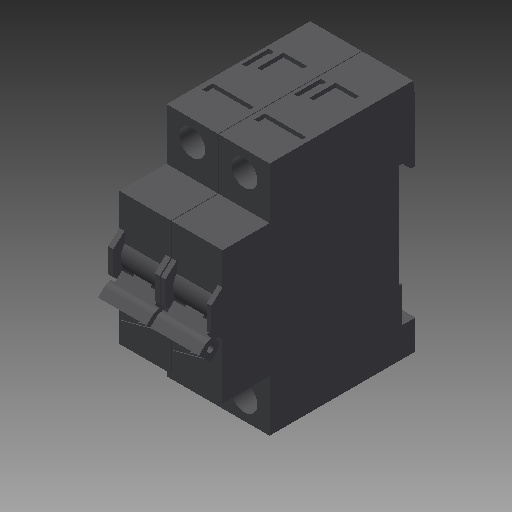
# Autodesk Inventor part: 278738
Saved by Autodesk Inventor 2019.3 (Build 233278000, 278)
## iProperties
Category: PARTsolutions
Company: MOELLER
Created: 2017-12-07
Part Number: 278738
Catalog Web Link: www.cadenas.de
Description: Miniature Circuit Breakers (MCBs)-
Vendor: MOELLER
Document SubType Name: Modeling
Designer: psAdmin
Manufacturer: MOELLER
Mass: 154.066 g
Surface Area: 233.199 cm^2
Volume: 154.066 cm^3
Density: 1 g/cm^3
Material: Типовые
Appearance: PSOLRGB-175-175-175
PSOL_IDENT_0: {$CADENAS_DATA\23d-libs\moeller\36899\36901\36903\36910.prj},196 {VTYP=3D},{NB=278738},{LINA=278738}
PSOL_IDENT_1: ,{NN=Miniature Circuit Breakers (MCBs)},{DATE=03.11.2017 09:05:45},{GEOMDATE=02.11.2017 14:51:53},{V
PSOL_IDENT_2: ERSION=v171102145153},{LINEID=8470},{LINESUBID=-1},{WBVAR=}  {NB=278738},{LINA=278738},{KT=DUMMY},{P
PSOL_IDENT_3: FOTO=sg55112.jpg},{PLID=278738},{DATA_SHEET=Data sheet},{MANUTYPEDESC=FAZ-B40/2},{DESCSHORT=Miniatur
PSOL_IDENT_4: e circuit breaker (MCB), 40A, 2p, B-Char, AC},{DESCLONG=Miniature circuit breaker (MCB) FAZ, 2 pole,
PSOL_IDENT_5: Tripping characteristic: B, Rated current In: 40 A, Switchgear for industrial and advanced commerci
PSOL_IDENT_6: al applications},{EAN=4015082787387},{ECLASS_8_1=27-14-19-01},{PACKAGED_WEIGHT=0.233},{DATA_SHEET_=h
PSOL_IDENT_7: ttp://datasheet.moeller.net/datasheet.php?model=278738&locale=en_GB},{DATA_SHEET_ENG=http://datashee
PSOL_IDENT_8: t.moeller.net/datasheet.php?model=278738&locale=en_GB},{DATA_SHEET_DEU=http://datasheet.moeller.net/
PSOL_IDENT_9: datasheet.php?model=278738&locale=de_DE}
NN: Miniature Circuit Breakers (MCBs)
NB: 278738
NBSYN: $PLID.
LINA: 278738
PFOTO: sg55112.jpg
PLID: 278738
DATA_SHEET: Data sheet
MANUTYPEDESC: FAZ-B40/2
DESCSHORT: Miniature circuit breaker (MCB), 40A, 2p, B-Char, AC
DESCLONG: Miniature circuit breaker (MCB) FAZ, 2 pole, Tripping characteristic: B, Rated current In: 40 A, Switchgear for industrial and advanced commercial applications
EAN: 4015082787387
ECLASS_8_1: 27-14-19-01
PACKAGED_WEIGHT: 0.233
SUPPLIER: MOELLER
ARTICLENO: 278738
BOMINFO: 278738
CREATOR: CADENAS GmbH
Title: 278738
Author: Cadenas PARTsolutions
Autodesk Inventor part; units mm, degrees
ref_plane "YZ Plane" through (0, 0, 0) normal (1, 0, 0) x (0, 1, 0)
ref_plane "XZ Plane" through (0, 0, 0) normal (0, 1, 0) x (-1, 0, 0)
ref_plane "XY Plane" through (0, 0, 0) normal (0, 0, 1) x (1, 0, 0)
sketch "Sketch_1" plane through (8.75, 0, 0) normal (1, 0, 0) x (0, 0, -1)
  line L0 (-63.8, 8.1) -> (-63.8, -0.1)
  line L1 (-63.8, -0.1) -> (-60, -3.6)
  line L2 (-60, -3.6) -> (-60, -22.5)
  line L3 (-60, -22.5) -> (-44, -22.5)
  line L4 (-44, -22.5) -> (-44, -40)
  line L5 (-44, -40) -> (5.5, -40)
  line L6 (5.5, -40) -> (5.5, -30)
  line L7 (5.5, -30) -> (1, -30)
  line L8 (1, -30) -> (1, -18.1)
  arc A0 (1, -18.1) -> (0.7, -17.8) centre (0.7, -18.1) ccw
  line L9 (0.7, -17.8) -> (0, -17.8)
  line L10 (0, -17.8) -> (0, 17.5)
  line L11 (0, 17.5) -> (1, 17.5)
  line L12 (1, 17.5) -> (4, 14.5)
  line L13 (4, 14.5) -> (5.5, 14.5)
  line L14 (5.5, 14.5) -> (5.5, 34)
  line L15 (5.5, 34) -> (4.7633, 40)
  line L16 (4.7633, 40) -> (-44, 40)
  line L17 (-44, 40) -> (-44, 22.5)
  line L18 (-44, 22.5) -> (-60, 22.5)
  line L19 (-60, 22.5) -> (-60, 11.6)
  line L20 (-60, 11.6) -> (-63.8, 8.1)
  constraints: 42 end point, 2 point on circle, 1 centre point
extrude "Extrusion1" add sketch "Sketch_1" along normal mid plane 17.5
sketch "Sketch_5" plane through (0, 0, 0) normal (0, 1, 0) x (-1, 0, 0)
  line L0 (-1.05, 19.5) -> (-2.9801, 19.5)
  line L1 (-2.9801, 19.5) -> (-2.9801, 10.4)
  line L2 (-2.9801, 10.4) -> (-1.05, 10.4)
  line L3 (-1.05, 10.4) -> (-1.05, 19.5)
  constraints: 8 end point
extrude "Extrusion2" cut sketch "Sketch_5" along normal mid plane 100
sketch "Sketch_6" plane through (0, 0, 0) normal (0, 1, 0) x (-1, 0, 0)
  line L0 (-4.75, 18) -> (-12.75, 18)
  line L1 (-12.75, 18) -> (-12.75, 9)
  line L2 (-12.75, 9) -> (-4.75, 9)
  line L3 (-4.75, 9) -> (-4.75, 18)
  constraints: 8 end point
extrude "Extrusion3" cut sketch "Sketch_6" along normal mid plane 100
sketch "Sketch_7" plane through (0, 0, 0) normal (0, 1, 0) x (-1, 0, 0)
  line L0 (-1.75, 33.6) -> (-15.75, 33.6)
  line L1 (-15.75, 33.6) -> (-15.75, 30)
  line L2 (-15.75, 30) -> (-1.75, 30)
  line L3 (-1.75, 30) -> (-1.75, 33.6)
  constraints: 8 end point
extrude "Extrusion4" cut sketch "Sketch_7" along normal mid plane 100
sketch "Sketch_8" plane through (0, 0, 0) normal (0, 1, 0) x (-1, 0, 0)
  line L0 (-0.75, 38) -> (-16.25, 38)
  line L1 (-16.25, 38) -> (-16.25, 8)
  line L2 (-16.25, 8) -> (-0.75, 8)
  line L3 (-0.75, 8) -> (-0.75, 38)
  constraints: 8 end point
extrude "Extrusion5" add sketch "Sketch_8" along normal mid plane 77.2
sketch "Sketch_19" plane through (0, 0, 60) normal (0, 0, 1) x (1, 0, 0)
  line L0 (0.05, -15.4982) -> (14.2251, -11.7)
  line L1 (14.2251, -11.7) -> (0.05, -7.9018)
  line L2 (0.05, -7.9018) -> (0.05, -15.4982)
  constraints: 6 end point
extrude "Extrusion6" cut sketch "Sketch_19" along normal mid plane 0.6
sketch "Sketch_20" plane through (0, 0, 60) normal (0, 0, 1) x (1, 0, 0)
  line L0 (5.95, -13.3345) -> (12.05, -11.7)
  line L1 (12.05, -11.7) -> (5.95, -10.0655)
  line L2 (5.95, -10.0655) -> (5.95, -13.3345)
  constraints: 6 end point
extrude "Extrusion7" cut sketch "Sketch_20" against normal blind 0.8
sketch "Sketch_22" plane through (26.45, 0, 0) normal (1, 0, 0) x (0, 0, -1)
  line L0 (-59.8, -22.3) -> (-43.8, -22.3)
  line L1 (-43.8, -22.3) -> (-43.8, -39.8)
  line L2 (-43.8, -39.8) -> (5.3, -39.8)
  line L3 (5.3, -39.8) -> (5.3, -30.2)
  line L4 (5.3, -30.2) -> (0.8, -30.2)
  line L5 (0.8, -30.2) -> (0.8, -18.3)
  arc A0 (0.8, -18.3) -> (0.5, -18) centre (0.5, -18.3) ccw
  line L6 (0.5, -18) -> (-0.2, -18)
  line L7 (-0.2, -18) -> (-0.2, 17.7)
  line L8 (-0.2, 17.7) -> (1, 17.7)
  line L9 (1, 17.7) -> (4, 14.7)
  line L10 (4, 14.7) -> (5.3, 14.7)
  line L11 (5.3, 14.7) -> (5.3, 34)
  line L12 (5.3, 34) -> (4.5878, 39.8)
  line L13 (4.5878, 39.8) -> (-43.8, 39.8)
  line L14 (-43.8, 39.8) -> (-43.8, 22.3)
  line L15 (-43.8, 22.3) -> (-59.8, 22.3)
  line L16 (-59.8, 22.3) -> (-59.8, -22.3)
  constraints: 34 end point, 2 point on circle, 1 centre point
extrude "Extrusion8" add sketch "Sketch_22" against normal blind 9
sketch "Sketch_24" plane through (26.45, 0, 0) normal (1, 0, 0) x (0, 0, -1)
  line L0 (-63.8, 8.1) -> (-63.8, -0.1)
  line L1 (-63.8, -0.1) -> (-60, -3.6)
  line L2 (-60, -3.6) -> (-60, -22.5)
  line L3 (-60, -22.5) -> (-44, -22.5)
  line L4 (-44, -22.5) -> (-44, -40)
  line L5 (-44, -40) -> (5.5, -40)
  line L6 (5.5, -40) -> (5.5, -30)
  line L7 (5.5, -30) -> (1, -30)
  line L8 (1, -30) -> (1, -18.1)
  arc A0 (1, -18.1) -> (0.7, -17.8) centre (0.7, -18.1) ccw
  line L9 (0.7, -17.8) -> (0, -17.8)
  line L10 (0, -17.8) -> (0, 17.5)
  line L11 (0, 17.5) -> (1, 17.5)
  line L12 (1, 17.5) -> (4, 14.5)
  line L13 (4, 14.5) -> (5.5, 14.5)
  line L14 (5.5, 14.5) -> (5.5, 34)
  line L15 (5.5, 34) -> (4.7633, 40)
  line L16 (4.7633, 40) -> (-44, 40)
  line L17 (-44, 40) -> (-44, 22.5)
  line L18 (-44, 22.5) -> (-60, 22.5)
  line L19 (-60, 22.5) -> (-60, 11.6)
  line L20 (-60, 11.6) -> (-63.8, 8.1)
  constraints: 42 end point, 2 point on circle, 1 centre point
extrude "Extrusion9" add sketch "Sketch_24" along normal mid plane 17.1
sketch "Sketch_28" plane through (0, 0, 0) normal (0, 1, 0) x (-1, 0, 0)
  line L0 (-18.75, 19.5) -> (-20.6801, 19.5)
  line L1 (-20.6801, 19.5) -> (-20.6801, 10.4)
  line L2 (-20.6801, 10.4) -> (-18.75, 10.4)
  line L3 (-18.75, 10.4) -> (-18.75, 19.5)
  constraints: 8 end point
extrude "Extrusion10" cut sketch "Sketch_28" along normal mid plane 100
sketch "Sketch_29" plane through (0, 0, 0) normal (0, 1, 0) x (-1, 0, 0)
  line L0 (-22.45, 18) -> (-30.45, 18)
  line L1 (-30.45, 18) -> (-30.45, 9)
  line L2 (-30.45, 9) -> (-22.45, 9)
  line L3 (-22.45, 9) -> (-22.45, 18)
  constraints: 8 end point
extrude "Extrusion11" cut sketch "Sketch_29" along normal mid plane 100
sketch "Sketch_30" plane through (0, 0, 0) normal (0, 1, 0) x (-1, 0, 0)
  line L0 (-19.45, 33.6) -> (-33.45, 33.6)
  line L1 (-33.45, 33.6) -> (-33.45, 30)
  line L2 (-33.45, 30) -> (-19.45, 30)
  line L3 (-19.45, 30) -> (-19.45, 33.6)
  constraints: 8 end point
extrude "Extrusion12" cut sketch "Sketch_30" along normal mid plane 100
sketch "Sketch_31" plane through (0, 0, 0) normal (0, 1, 0) x (-1, 0, 0)
  line L0 (-18.25, 38) -> (-33.75, 38)
  line L1 (-33.75, 38) -> (-33.75, 8)
  line L2 (-33.75, 8) -> (-18.25, 8)
  line L3 (-18.25, 8) -> (-18.25, 38)
  constraints: 8 end point
extrude "Extrusion13" add sketch "Sketch_31" along normal mid plane 77.2
sketch "Sketch_13" plane through (0, 0, 0) normal (0, 1, 0) x (-1, 0, 0)
  line L0 (15.95, 70) -> (-33.45, 70)
  line L1 (-33.45, 70) -> (-33.45, 60)
  line L2 (-33.45, 60) -> (-19.45, 60)
  line L3 (-19.45, 60) -> (-19.45, 65)
  line L4 (-19.45, 65) -> (-15.75, 65)
  line L5 (-15.75, 65) -> (-15.75, 60)
  line L6 (-15.75, 60) -> (-1.75, 60)
  line L7 (-1.75, 60) -> (-1.75, 65)
  line L8 (-1.75, 65) -> (1.95, 65)
  line L9 (1.95, 65) -> (1.95, 60)
  line L10 (1.95, 60) -> (15.95, 60)
  line L11 (15.95, 60) -> (15.95, 70)
  constraints: 24 end point
extrude "Extrusion14" cut sketch "Sketch_13" along normal mid plane 40
sketch "Sketch_14" plane through (8.75, 0, 0) normal (1, 0, 0) x (0, 0, -1)
  circle A0 centre (-55, 4) radius 6.35
  constraints: 1 centre point
extrude "Extrusion15" add sketch "Sketch_14" along normal mid plane 14
sketch "Sketch_15" plane through (26.45, 0, 0) normal (1, 0, 0) x (0, 0, -1)
  circle A0 centre (-55, 4) radius 6.35
  constraints: 1 centre point
extrude "Extrusion16" add sketch "Sketch_15" along normal mid plane 14
sketch "Sketch_17" plane through (8.75, 0, 0) normal (1, 0, 0) x (0, 0, -1)
  line L0 (-63.6974, -1.869) -> (-60.8581, -4.7082)
  line L1 (-60.8581, -4.7082) -> (-57.6762, -1.5262)
  line L2 (-57.6762, -1.5262) -> (-60.5154, 1.313)
  line L3 (-60.5154, 1.313) -> (-63.6974, -1.869)
  constraints: 8 end point
extrude "Extrusion17" add sketch "Sketch_17" along normal mid plane 6
sketch "Sketch_18" plane through (8.75, 0, 0) normal (1, 0, 0) x (0, 0, -1)
  line L0 (-63.6974, -1.869) -> (-60.8581, -4.7082)
  line L1 (-60.8581, -4.7082) -> (-58.3126, -2.1626)
  line L2 (-58.3126, -2.1626) -> (-61.1518, 0.6766)
  line L3 (-61.1518, 0.6766) -> (-63.6974, -1.869)
  constraints: 8 end point
extrude "Extrusion18" add sketch "Sketch_18" along normal mid plane 13.5
sketch "Sketch_33" plane through (8.75, 0, 0) normal (1, 0, 0) x (0, 0, -1)
  line L0 (-67.7279, -4.7681) -> (-63.7681, -8.7279)
  line L1 (-63.7681, -8.7279) -> (-61.7882, -6.748)
  arc A0 (-61.7882, -6.748) -> (-60.9686, -4.8186) centre (-63.7681, -4.7681) ccw
  line L2 (-60.9686, -4.8186) -> (-60.6039, -4.454)
  line L3 (-60.6039, -4.454) -> (-63.4431, -1.6147)
  line L4 (-63.4431, -1.6147) -> (-63.7966, -1.9682)
  arc A1 (-63.7966, -1.9682) -> (-65.748, -2.7882) centre (-63.7681, -4.7681) ccw
  line L5 (-65.748, -2.7882) -> (-67.7279, -4.7681)
  constraints: 12 end point, 4 point on circle, 2 centre point
extrude "Extrusion19" add sketch "Sketch_33" along normal mid plane 16.5
sketch "Sketch_36" plane through (0, 0, 60) normal (0, 0, 1) x (1, 0, 0)
  line L0 (17.7, -15.4982) -> (31.8751, -11.7)
  line L1 (31.8751, -11.7) -> (17.7, -7.9018)
  line L2 (17.7, -7.9018) -> (17.7, -15.4982)
  constraints: 6 end point
extrude "Extrusion20" cut sketch "Sketch_36" along normal mid plane 0.6
sketch "Sketch_37" plane through (0, 0, 60) normal (0, 0, 1) x (1, 0, 0)
  line L0 (23.65, -13.3345) -> (29.75, -11.7)
  line L1 (29.75, -11.7) -> (23.65, -10.0655)
  line L2 (23.65, -10.0655) -> (23.65, -13.3345)
  constraints: 6 end point
extrude "Extrusion21" cut sketch "Sketch_37" against normal blind 0.8
sketch "Sketch_39" plane through (26.45, 0, 0) normal (1, 0, 0) x (0, 0, -1)
  line L0 (-63.6974, -1.869) -> (-60.8581, -4.7082)
  line L1 (-60.8581, -4.7082) -> (-57.6762, -1.5262)
  line L2 (-57.6762, -1.5262) -> (-60.5154, 1.313)
  line L3 (-60.5154, 1.313) -> (-63.6974, -1.869)
  constraints: 8 end point
extrude "Extrusion22" add sketch "Sketch_39" along normal mid plane 6
sketch "Sketch_41" plane through (26.45, 0, 0) normal (1, 0, 0) x (0, 0, -1)
  line L0 (-63.6974, -1.869) -> (-60.8581, -4.7082)
  line L1 (-60.8581, -4.7082) -> (-58.3126, -2.1626)
  line L2 (-58.3126, -2.1626) -> (-61.1518, 0.6766)
  line L3 (-61.1518, 0.6766) -> (-63.6974, -1.869)
  constraints: 8 end point
extrude "Extrusion23" add sketch "Sketch_41" along normal mid plane 13.5
sketch "Sketch_43" plane through (26.45, 0, 0) normal (1, 0, 0) x (0, 0, -1)
  line L0 (-67.7279, -4.7681) -> (-63.7681, -8.7279)
  line L1 (-63.7681, -8.7279) -> (-61.7882, -6.748)
  arc A0 (-61.7882, -6.748) -> (-60.9686, -4.8186) centre (-63.7681, -4.7681) ccw
  line L2 (-60.9686, -4.8186) -> (-60.6039, -4.454)
  line L3 (-60.6039, -4.454) -> (-63.4431, -1.6147)
  line L4 (-63.4431, -1.6147) -> (-63.7966, -1.9682)
  arc A1 (-63.7966, -1.9682) -> (-65.748, -2.7882) centre (-63.7681, -4.7681) ccw
  line L5 (-65.748, -2.7882) -> (-67.7279, -4.7681)
  constraints: 12 end point, 4 point on circle, 2 centre point
extrude "Extrusion24" add sketch "Sketch_43" along normal mid plane 16.5
sketch "Sketch_44" plane through (8.75, 0, 0) normal (1, 0, 0) x (0, 0, -1)
  circle A0 centre (-63.7681, -4.7681) radius 1.11
  constraints: 1 centre point
extrude "Extrusion25" cut sketch "Sketch_44" along normal mid plane 100
sketch "Sketch_45_ALT_Drilling_1" plane through (0, 0, 44) normal (0, 0, 1) x (1, 0, 0)
  circle A0 centre (8.75, 33) radius 4.4
  constraints: 1 centre point
extrude "Extrusion26" cut sketch "Sketch_45_ALT_Drilling_1" against normal blind 9
sketch "Sketch_12_ALT_Drilling_2" plane through (0, 0, 44) normal (0, 0, 1) x (1, 0, 0)
  circle A0 centre (26.45, 33) radius 4.4
  constraints: 1 centre point
extrude "Extrusion27" cut sketch "Sketch_12_ALT_Drilling_2" against normal blind 9
sketch "Sketch_16_ALT_Drilling_3" plane through (0, 0, 44) normal (0, 0, 1) x (1, 0, 0)
  circle A0 centre (8.75, -33) radius 4.4
  constraints: 1 centre point
extrude "Extrusion28" cut sketch "Sketch_16_ALT_Drilling_3" against normal blind 9
sketch "Sketch_21_ALT_Drilling_4" plane through (0, 0, 44) normal (0, 0, 1) x (1, 0, 0)
  circle A0 centre (26.45, -33) radius 4.4
  constraints: 1 centre point
extrude "Extrusion29" cut sketch "Sketch_21_ALT_Drilling_4" against normal blind 9
sketch "Sketch_47" plane through (0, 0, 44) normal (0, 0, 1) x (1, 0, 0)
  line L0 (5.4414, 35.2479) -> (7.6893, 33)
  line L1 (7.6893, 33) -> (6.5333, 31.844)
  arc A0 (6.5333, 31.844) -> (7.594, 30.7833) centre (8.75, 33) ccw
  line L2 (7.594, 30.7833) -> (8.75, 31.9393)
  line L3 (8.75, 31.9393) -> (10.9979, 29.6914)
  arc A1 (10.9979, 29.6914) -> (12.0586, 30.7521) centre (8.75, 33) ccw
  line L4 (12.0586, 30.7521) -> (9.8107, 33)
  line L5 (9.8107, 33) -> (10.9667, 34.156)
  arc A2 (10.9667, 34.156) -> (9.906, 35.2167) centre (8.75, 33) ccw
  line L6 (9.906, 35.2167) -> (8.75, 34.0607)
  line L7 (8.75, 34.0607) -> (6.5021, 36.3086)
  arc A3 (6.5021, 36.3086) -> (5.4414, 35.2479) centre (8.75, 33) ccw
  constraints: 16 end point, 8 point on circle, 4 centre point
extrude "Extrusion30" cut sketch "Sketch_47" against normal blind 10.6
sketch "Sketch_23" plane through (0, 0, 44) normal (0, 0, 1) x (1, 0, 0)
  line L0 (23.1414, 35.2479) -> (25.3893, 33)
  line L1 (25.3893, 33) -> (24.2333, 31.844)
  arc A0 (24.2333, 31.844) -> (25.294, 30.7833) centre (26.45, 33) ccw
  line L2 (25.294, 30.7833) -> (26.45, 31.9393)
  line L3 (26.45, 31.9393) -> (28.6979, 29.6914)
  arc A1 (28.6979, 29.6914) -> (29.7586, 30.7521) centre (26.45, 33) ccw
  line L4 (29.7586, 30.7521) -> (27.5107, 33)
  line L5 (27.5107, 33) -> (28.6667, 34.156)
  arc A2 (28.6667, 34.156) -> (27.606, 35.2167) centre (26.45, 33) ccw
  line L6 (27.606, 35.2167) -> (26.45, 34.0607)
  line L7 (26.45, 34.0607) -> (24.2021, 36.3086)
  arc A3 (24.2021, 36.3086) -> (23.1414, 35.2479) centre (26.45, 33) ccw
  constraints: 16 end point, 8 point on circle, 4 centre point
extrude "Extrusion31" cut sketch "Sketch_23" against normal blind 10.6
sketch "Sketch_25" plane through (0, 0, 44) normal (0, 0, 1) x (1, 0, 0)
  line L0 (5.4414, -30.7521) -> (7.6893, -33)
  line L1 (7.6893, -33) -> (6.5333, -34.156)
  arc A0 (6.5333, -34.156) -> (7.594, -35.2167) centre (8.75, -33) ccw
  line L2 (7.594, -35.2167) -> (8.75, -34.0607)
  line L3 (8.75, -34.0607) -> (10.9979, -36.3086)
  arc A1 (10.9979, -36.3086) -> (12.0586, -35.2479) centre (8.75, -33) ccw
  line L4 (12.0586, -35.2479) -> (9.8107, -33)
  line L5 (9.8107, -33) -> (10.9667, -31.844)
  arc A2 (10.9667, -31.844) -> (9.906, -30.7833) centre (8.75, -33) ccw
  line L6 (9.906, -30.7833) -> (8.75, -31.9393)
  line L7 (8.75, -31.9393) -> (6.5021, -29.6914)
  arc A3 (6.5021, -29.6914) -> (5.4414, -30.7521) centre (8.75, -33) ccw
  constraints: 16 end point, 8 point on circle, 4 centre point
extrude "Extrusion32" cut sketch "Sketch_25" against normal blind 10.6
sketch "Sketch_26" plane through (0, 0, 44) normal (0, 0, 1) x (1, 0, 0)
  line L0 (23.1414, -30.7521) -> (25.3893, -33)
  line L1 (25.3893, -33) -> (24.2333, -34.156)
  arc A0 (24.2333, -34.156) -> (25.294, -35.2167) centre (26.45, -33) ccw
  line L2 (25.294, -35.2167) -> (26.45, -34.0607)
  line L3 (26.45, -34.0607) -> (28.6979, -36.3086)
  arc A1 (28.6979, -36.3086) -> (29.7586, -35.2479) centre (26.45, -33) ccw
  line L4 (29.7586, -35.2479) -> (27.5107, -33)
  line L5 (27.5107, -33) -> (28.6667, -31.844)
  arc A2 (28.6667, -31.844) -> (27.606, -30.7833) centre (26.45, -33) ccw
  line L6 (27.606, -30.7833) -> (26.45, -31.9393)
  line L7 (26.45, -31.9393) -> (24.2021, -29.6914)
  arc A3 (24.2021, -29.6914) -> (23.1414, -30.7521) centre (26.45, -33) ccw
  constraints: 16 end point, 8 point on circle, 4 centre point
extrude "Extrusion33" cut sketch "Sketch_26" against normal blind 10.6
sketch "Sketch_3" plane through (8.75, 0, 0) normal (1, 0, 0) x (0, 0, -1)
  line L0 (1.075, -16.4252) -> (1.075, -44.7)
  line L1 (1.075, -44.7) -> (3.875, -44.7)
  line L2 (3.875, -44.7) -> (3.875, -16.728)
  line L3 (3.875, -16.728) -> (1.575, -15.4001)
  line L4 (1.575, -15.4001) -> (1.075, -16.4252)
  constraints: 10 end point
extrude "Extrusion34" add sketch "Sketch_3" along normal mid plane 11
sketch "Sketch_4" plane through (8.75, 0, 0) normal (1, 0, 0) x (0, 0, -1)
  line L0 (-0.075, -18.9) -> (5.475, -18.9)
  line L1 (5.475, -18.9) -> (5.475, -17.6518)
  line L2 (5.475, -17.6518) -> (1.575, -15.4001)
  line L3 (1.575, -15.4001) -> (0.7215, -17.15)
  line L4 (0.7215, -17.15) -> (-0.075, -17.15)
  line L5 (-0.075, -17.15) -> (-0.075, -18.9)
  constraints: 12 end point
extrude "Extrusion35" add sketch "Sketch_4" along normal mid plane 4
sketch "Sketch_9" plane through (0, 0, 0) normal (0, 0, 1) x (1, 0, 0)
  arc A0 (5.5, -41.95) -> (6.25, -42.7) centre (6.25, -41.95) ccw
  line L0 (6.25, -42.7) -> (11.25, -42.7)
  arc A1 (11.25, -42.7) -> (12, -41.95) centre (11.25, -41.95) ccw
  line L1 (12, -41.95) -> (12, -41.3)
  arc A2 (12, -41.3) -> (11.7, -41) centre (11.7, -41.3) ccw
  line L2 (11.7, -41) -> (5.8, -41)
  arc A3 (5.8, -41) -> (5.5, -41.3) centre (5.8, -41.3) ccw
  line L3 (5.5, -41.3) -> (5.5, -41.95)
  constraints: 8 end point, 8 point on circle, 4 centre point
extrude "Extrusion36" cut sketch "Sketch_9" against normal blind 9.156
sketch "Sketch_2" plane through (0, 0, 0) normal (0, 0, 1) x (1, 0, 0)
  line L0 (-1.25, -50) -> (18.75, -50)
  line L1 (18.75, -50) -> (18.75, -40)
  line L2 (18.75, -40) -> (13.75, -40)
  line L3 (13.75, -40) -> (13.75, -47)
  line L4 (13.75, -47) -> (3.75, -47)
  line L5 (3.75, -47) -> (3.75, -40)
  line L6 (3.75, -40) -> (-1.25, -40)
  line L7 (-1.25, -40) -> (-1.25, -50)
  constraints: 16 end point
extrude "Extrusion37" cut sketch "Sketch_2" against normal blind 9.156
sketch "Sketch_10" plane through (17.5, 0, 0) normal (1, 0, 0) x (0, 0, -1)
  circle A0 centre (-63.7681, -4.7681) radius 1.11
  constraints: 1 centre point
extrude "Extrusion38" add sketch "Sketch_10" along normal mid plane 25.2
sketch "Sketch_11" plane through (0, 0, 0) normal (0, 1, 0) x (-1, 0, 0)
  line L0 (-20.8, -1.075) -> (-32, -1.075)
  line L1 (-32, -1.075) -> (-32, -3.875)
  line L2 (-32, -3.875) -> (-20.8, -3.875)
  line L3 (-20.8, -3.875) -> (-20.8, -1.075)
  constraints: 8 end point
extrude "Extrusion39" cut sketch "Sketch_11" against normal blind 50
body "Solid1"
